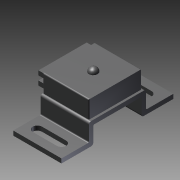
# Autodesk Inventor part: HMEN5-5-magnet
Saved by Autodesk Inventor 2015 SP1 (Build 190203100, 203)
## iProperties
Category: Hardware
Company: MISUMI
Created: 2015-02-01
Part Number: HMEN5-5-magnet
Catalog Web Link: http://us.misumi-ec.com/vona2/detail/110300479530
Description: HMEN, HMER-magnet-Latch Magnets for Plate
Vendor: MISUMI
Document SubType Name: Modeling
Designer: psAdmin
Manufacturer: MISUMI
Mass: 7.00245 g
Surface Area: 41.5138 cm^2
Volume: 7.00245 cm^3
Density: 1 g/cm^3
Material: Generic
Appearance: PSOLRGB-192-192-192
PSOL_IDENT_0: {\\10.0.0.236\data_v8\23d-libs\misumi\metric\39_accessories_for_al_extrusions\hmen_magnet.prj},183 {
PSOL_IDENT_1: VTYP=3D},{NB=HMEN5-5-magnet},{LINA=HMEN5-5-magnet},{NN=HMEN, HMER-magnet},{DATE=17.11.2014 05:31:12}
PSOL_IDENT_2: ,{GEOMDATE=08.06.2009 12:14:00},{VERSION=},{LINEID=10},{LINESUBID=-1},{WBVAR=TS}  {NB=HMEN5-5-magnet
PSOL_IDENT_3: },{LINA=HMEN5-5-magnet},{KT=DUMMY},{PN=HMEN5-5},{TYPE=HMEN},{TS=HMEN},{MAT=304 Stainless Steel},{ST=
PSOL_IDENT_4: Dark Brown Painting},{NO=5-5},{MAG=T Magnet},{HF=29.4 (3)},{AP=MG5-5},{AP1=-},{CSS=Truss Screw M4-5}
PSOL_IDENT_5: ,{QSS=2},{CB1=CBM5-25},{QB1=2},{CW=-},{QW=-},{CB2=-},{QB2=-},{CB3=-},{QB3=-},{CN1=HNTT5-5},{QN1=2},{
PSOL_IDENT_6: CFS=M3-6},{QFS=1},{CN2=HNTT5-3},{QN2=1},{APP=1},{M=4},{A=51},{B=20},{H=0},{L=0},{T=15.0},{G=31},{S=6
PSOL_IDENT_7: },{V=5.0},{Y=10},{E=0},{X=15},{F=0},{MMIN=3.242},{Z=12},{Z1=4},{P1=18},{PX=6},{PY=19.5},{EXT=3.000},
PSOL_IDENT_8: {TRANS=-1},{WAS=9.2},{X1=9.2},{YY=-2}
SUPPLIER: MISUMI
ARTICLENO: HMEN5-5-magnet
BOMINFO: HMEN5-5-magnet
CREATOR: CADENAS GmbH
Title: HMEN5-5-magnet
Author: Misumi
Comments: Latch Magnets for Plate
Autodesk Inventor part; units mm, degrees
ref_plane "YZ Plane" through (0, 0, 0) normal (1, 0, 0) x (0, 1, 0)
ref_plane "XZ Plane" through (0, 0, 0) normal (0, 1, 0) x (-1, 0, 0)
ref_plane "XY Plane" through (0, 0, 0) normal (0, 0, 1) x (1, 0, 0)
sketch "Sketch_1" plane through (0, 0, 0) normal (1, 0, 0) x (0, 1, 0)
  arc A0 (-11.5, 0) -> (-12, -0.5) centre (-11.5, -0.5) ccw
  line L0 (-12, -0.5) -> (-12, -8)
  arc A1 (-12, -8) -> (-13, -9) centre (-12, -9) ccw
  line L1 (-13, -9) -> (-13, -15.5)
  arc A2 (-13.5, -16) -> (-13, -15.5) centre (-13.5, -15.5) ccw
  line L2 (-13.5, -16) -> (-25.5, -16)
  line L3 (-25.5, -16) -> (-25.5, -18)
  line L4 (-25.5, -18) -> (-12, -18)
  arc A3 (-12, -18) -> (-11, -17) centre (-12, -17) ccw
  line L5 (-11, -17) -> (-11, -10.5)
  arc A4 (-10.5, -10) -> (-11, -10.5) centre (-10.5, -10.5) ccw
  line L6 (-10.5, -10) -> (10.5, -10)
  arc A5 (11, -10.5) -> (10.5, -10) centre (10.5, -10.5) ccw
  line L7 (11, -10.5) -> (11, -17)
  arc A6 (11, -17) -> (12, -18) centre (12, -17) ccw
  line L8 (12, -18) -> (25.5, -18)
  line L9 (25.5, -18) -> (25.5, -16)
  line L10 (25.5, -16) -> (13.5, -16)
  arc A7 (13, -15.5) -> (13.5, -16) centre (13.5, -15.5) ccw
  line L11 (13, -15.5) -> (13, -9)
  arc A8 (13, -9) -> (12, -8) centre (12, -9) ccw
  line L12 (12, -8) -> (12, -0.5)
  arc A9 (12, -0.5) -> (11.5, 0) centre (11.5, -0.5) ccw
  line L13 (11.5, 0) -> (-11.5, 0)
  constraints: 28 end point, 20 point on circle, 10 centre point
extrude "Extrusion1" add sketch "Sketch_1" along normal mid plane 22
sketch "Sketch_2" plane through (0, 0, 0) normal (0, 0, 1) x (1, 0, 0)
  line L0 (10, 12) -> (10, -12)
  line L1 (10, -12) -> (11, -12)
  line L2 (11, -12) -> (11, 12)
  line L3 (11, 12) -> (10, 12)
  constraints: 8 end point
extrude "Extrusion2" cut sketch "Sketch_2" against normal blind 8
sketch "Sketch_3" plane through (0, 0, 0) normal (0, 0, 1) x (1, 0, 0)
  line L0 (50, 0) -> (-50, 0)
  arc A0 (2, 0) -> (-2, 0) centre (0, 0) ccw
  line L1 (2, 0) -> (-2, 0)
  constraints: 4 end point, 2 point on circle, 1 centre point
revolve "Revolution1" add sketch "Sketch_3" angle 360 about axis through (50, 0, 0) along (1, 0, 0)
sketch "Sketch_6" plane through (0, 0, 0) normal (0, 0, 1) x (1, 0, 0)
  line L0 (-24, 24) -> (-24, -24)
  line L1 (-24, -24) -> (24, -24)
  line L2 (24, -24) -> (24, 24)
  line L3 (24, 24) -> (-24, 24)
  line L4 (-11, 11.5) -> (-11, -11.5)
  arc A0 (-11, -11.5) -> (-10.5, -12) centre (-10.5, -11.5) ccw
  line L5 (-10.5, -12) -> (9.5, -12)
  arc A1 (9.5, -12) -> (10, -11.5) centre (9.5, -11.5) ccw
  line L6 (10, -11.5) -> (10, 11.5)
  arc A2 (10, 11.5) -> (9.5, 12) centre (9.5, 11.5) ccw
  line L7 (9.5, 12) -> (-10.5, 12)
  arc A3 (-10.5, 12) -> (-11, 11.5) centre (-10.5, 11.5) ccw
  constraints: 16 end point, 8 point on circle, 4 centre point
extrude "Extrusion3" cut sketch "Sketch_6" against normal blind 8
sketch "Sketch_4" plane through (-11, 0, 0) normal (1, 0, 0) x (0, 0, -1)
  line L0 (1, 11) -> (1, -11)
  line L1 (1, -11) -> (3, -11)
  line L2 (3, -11) -> (3, 11)
  line L3 (3, 11) -> (1, 11)
  constraints: 8 end point
extrude "Extrusion4" add sketch "Sketch_4" against normal blind 3
sketch "Sketch_5" plane through (-11, 0, 0) normal (1, 0, 0) x (0, 0, -1)
  line L0 (5, -11) -> (7, -11)
  line L1 (7, -11) -> (7, 11)
  line L2 (7, 11) -> (5, 11)
  line L3 (5, 11) -> (5, -11)
  constraints: 8 end point
extrude "Extrusion5" add sketch "Sketch_5" against normal blind 3
sketch "Sketch_7" plane through (0, 0, 0) normal (0, 0, 1) x (1, 0, 0)
  arc A0 (-6, 21.6) -> (-6, 17.4) centre (-6, 19.5) ccw
  line L0 (-6, 17.4) -> (5, 17.4)
  arc A1 (5, 17.4) -> (5, 21.6) centre (5, 19.5) ccw
  line L1 (5, 21.6) -> (-6, 21.6)
  constraints: 4 end point, 4 point on circle, 2 centre point
extrude "Extrusion6" cut sketch "Sketch_7" against normal blind 20
sketch "Sketch_8" plane through (0, 0, 0) normal (0, 0, 1) x (1, 0, 0)
  arc A0 (-6, -17.4) -> (-6, -21.6) centre (-6, -19.5) ccw
  line L0 (-6, -21.6) -> (5, -21.6)
  arc A1 (5, -21.6) -> (5, -17.4) centre (5, -19.5) ccw
  line L1 (5, -17.4) -> (-6, -17.4)
  constraints: 4 end point, 4 point on circle, 2 centre point
extrude "Extrusion7" cut sketch "Sketch_8" against normal blind 20
ref_plane "magnet_dummy_XY" through (0, 0, 0) normal (0, 0, 1) x (1, 0, 0)
ref_plane "magnet_dummy_YZ" through (0, 0, 0) normal (1, 0, 0) x (0, 1, 0)
ref_plane "magnet_dummy_ZX" through (0, 0, 0) normal (0, 1, 0) x (0, 0, 1)
ref_plane "to_ap_plate_XY" through (-9.1, 26, 0) normal (0, 0, -1) x (1, 0, 0)
ref_plane "to_ap_plate_YZ" through (-9.1, 26, 0) normal (1, 0, 0) x (0, -1, 0)
ref_plane "to_ap_plate_ZX" through (-9.1, 26, 0) normal (0, -1, 0) x (0, 0, -1)
ref_plane "to_door_side_plate_XY" through (-14, 0, -6) normal (1, 0, 0) x (0, 0, -1)
ref_plane "to_door_side_plate_YZ" through (-14, 0, -6) normal (0, 0, -1) x (0, 1, 0)
ref_plane "to_door_side_plate_ZX" through (-14, 0, -6) normal (0, 1, 0) x (1, 0, 0)
ref_plane "to_ap_plate1_XY" through (-1, 19.5, -18) normal (0, 0, 1) x (1, 0, 0)
ref_plane "to_ap_plate1_YZ" through (-1, 19.5, -18) normal (1, 0, 0) x (0, 1, 0)
ref_plane "to_ap_plate1_ZX" through (-1, 19.5, -18) normal (0, 1, 0) x (0, 0, 1)
ref_plane "to_ap_plate2_XY" through (-1, -19.5, -18) normal (0, 0, 1) x (1, 0, 0)
ref_plane "to_ap_plate2_YZ" through (-1, -19.5, -18) normal (1, 0, 0) x (0, 1, 0)
ref_plane "to_ap_plate2_ZX" through (-1, -19.5, -18) normal (0, 1, 0) x (0, 0, 1)
ref_plane "x1_XY" through (-9.2, 26, -15) normal (0, 0, -1) x (1, 0, 0)
ref_plane "x1_YZ" through (-9.2, 26, -15) normal (1, 0, 0) x (0, -1, 0)
ref_plane "x1_ZX" through (-9.2, 26, -15) normal (0, -1, 0) x (0, 0, -1)
ref_plane "x2_XY" through (-9.2, -26, -15) normal (0, 0, -1) x (1, 0, 0)
ref_plane "x2_YZ" through (-9.2, -26, -15) normal (1, 0, 0) x (0, -1, 0)
ref_plane "x2_ZX" through (-9.2, -26, -15) normal (0, -1, 0) x (0, 0, -1)
ref_plane "magnet_to_dummy2_XY" through (0, 0, -15) normal (0, 0, 1) x (1, 0, 0)
ref_plane "magnet_to_dummy2_YZ" through (0, 0, -15) normal (1, 0, 0) x (0, 1, 0)
ref_plane "magnet_to_dummy2_ZX" through (0, 0, -15) normal (0, 1, 0) x (0, 0, 1)
ref_plane "xy1_XY" through (-9.5, -26, 0) normal (0, 0, 1) x (1, 0, 0)
ref_plane "xy1_YZ" through (-9.5, -26, 0) normal (1, 0, 0) x (0, 1, 0)
ref_plane "xy1_ZX" through (-9.5, -26, 0) normal (0, 1, 0) x (0, 0, 1)
ref_plane "x22_XY" through (-9.1, -26, -7.5) normal (0, 0, -1) x (1, 0, 0)
ref_plane "x22_YZ" through (-9.1, -26, -7.5) normal (1, 0, 0) x (0, -1, 0)
ref_plane "x22_ZX" through (-9.1, -26, -7.5) normal (0, -1, 0) x (0, 0, -1)
ref_plane "to_ap_platexxx_XY" through (-9.1, 26, 0) normal (0, 0, -1) x (1, 0, 0)
ref_plane "to_ap_platexxx_YZ" through (-9.1, 26, 0) normal (1, 0, 0) x (0, -1, 0)
ref_plane "to_ap_platexxx_ZX" through (-9.1, 26, 0) normal (0, -1, 0) x (0, 0, -1)
ref_plane "to_ap_plate3_XY" through (-1, -19.5, -18) normal (0, 0, 1) x (1, 0, 0)
ref_plane "to_ap_plate3_YZ" through (-1, -19.5, -18) normal (1, 0, 0) x (0, 1, 0)
ref_plane "to_ap_plate3_ZX" through (-1, -19.5, -18) normal (0, 1, 0) x (0, 0, 1)
ref_plane "magnet_to_plate_XY" through (0, 19.5, -18) normal (1, 0, 0) x (0, 0, -1)
ref_plane "magnet_to_plate_YZ" through (0, 19.5, -18) normal (0, 0, -1) x (0, 1, 0)
ref_plane "magnet_to_plate_ZX" through (0, 19.5, -18) normal (0, 1, 0) x (1, 0, 0)
ref_plane "to_plate_XY" through (-9.1, 26, -15) normal (0, 0, -1) x (1, 0, 0)
ref_plane "to_plate_YZ" through (-9.1, 26, -15) normal (1, 0, 0) x (0, -1, 0)
ref_plane "to_plate_ZX" through (-9.1, 26, -15) normal (0, -1, 0) x (0, 0, -1)
ref_plane "to_pwf_bolt_XY" through (-9.1, 26, 0) normal (0, 0, -1) x (1, 0, 0)
ref_plane "to_pwf_bolt_YZ" through (-9.1, 26, 0) normal (1, 0, 0) x (0, -1, 0)
ref_plane "to_pwf_bolt_ZX" through (-9.1, 26, 0) normal (0, -1, 0) x (0, 0, -1)
ref_plane "to_pwf_bolt_1_XY" through (-9.1, -26, 0) normal (0, 0, -1) x (1, 0, 0)
ref_plane "to_pwf_bolt_1_YZ" through (-9.1, -26, 0) normal (1, 0, 0) x (0, -1, 0)
ref_plane "to_pwf_bolt_1_ZX" through (-9.1, -26, 0) normal (0, -1, 0) x (0, 0, -1)
ref_plane "washer_1_XY" through (-9.2, 26, 0) normal (0, 0, -1) x (1, 0, 0)
ref_plane "washer_1_YZ" through (-9.2, 26, 0) normal (1, 0, 0) x (0, -1, 0)
ref_plane "washer_1_ZX" through (-9.2, 26, 0) normal (0, -1, 0) x (0, 0, -1)
ref_plane "washer_2_XY" through (-9.2, -26, 0) normal (0, 0, -1) x (1, 0, 0)
ref_plane "washer_2_YZ" through (-9.2, -26, 0) normal (1, 0, 0) x (0, -1, 0)
ref_plane "washer_2_ZX" through (-9.2, -26, 0) normal (0, -1, 0) x (0, 0, -1)
ref_plane "pmf_1_XY" through (-9.2, 26, 0.8) normal (0, 0, -1) x (1, 0, 0)
ref_plane "pmf_1_YZ" through (-9.2, 26, 0.8) normal (1, 0, 0) x (0, -1, 0)
ref_plane "pmf_1_ZX" through (-9.2, 26, 0.8) normal (0, -1, 0) x (0, 0, -1)
ref_plane "pmf_2_XY" through (-9.2, -26, 0.8) normal (0, 0, -1) x (1, 0, 0)
ref_plane "pmf_2_YZ" through (-9.2, -26, 0.8) normal (1, 0, 0) x (0, -1, 0)
ref_plane "pmf_2_ZX" through (-9.2, -26, 0.8) normal (0, -1, 0) x (0, 0, -1)
body "Solid1"
